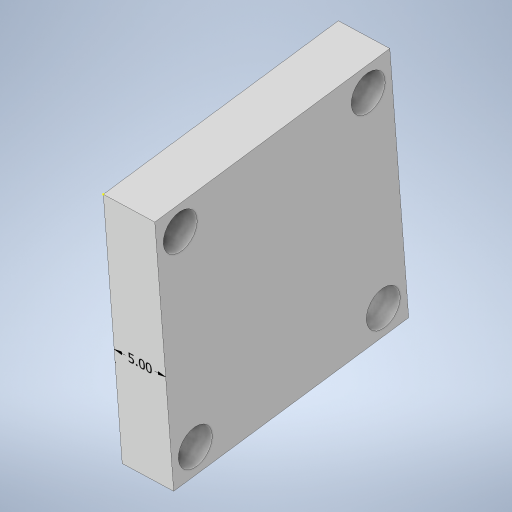
# Autodesk Inventor part: Plate_5mmforPrint
Saved by Autodesk Inventor 2024 (Build 280153000, 153)
## iProperties
Created: 2023-11-01
Part Number: Plate_5mmforPrint
Material: 一般
Document SubType Name: Modeling
Designer: jwith
Density: 1 g/cm^3
Appearance: 既定
Author: jwith
Autodesk Inventor part; units mm, degrees
ref_plane "YZ Plane" through (0, 0, 0) normal (1, 0, 0) x (0, 1, 0)
ref_plane "XZ Plane" through (0, 0, 0) normal (0, 1, 0) x (-1, 0, 0)
ref_plane "XY Plane" through (0, 0, 0) normal (0, 0, 1) x (1, 0, 0)
sketch "スケッチ1" plane through (0, 0, 0) normal (0, 1, 0) x (-1, 0, 0)
  line L0 (0, 0) -> (25, 0)
  line L1 (25, 0) -> (25, -25)
  line L2 (25, -25) -> (0, -25)
  line L3 (0, -25) -> (0, 0)
  dimension "d0" = 25
  dimension "d1" = 25
  constraints: 8 end point, 2 parallel, 1 horizontal, 1 perpendicular
  measures "d0" distance of L0.end L1.end
  measures "d1" distance of L1.end L2.end
extrude "押し出し1" add sketch "スケッチ1" against normal blind 5
sketch "スケッチ2" plane through (0, 0, 0) normal (0, 1, 0) x (1, 0, 0)
  line L0 (0, 25) -> (-25, 25) projected
  line L1 (0, 0) -> (0, 25) projected
  point P0 (-2.5, 22.5)
  point P1 (-22.5, 22.5)
  point P2 (-22.5, 2.5)
  point P3 (-2.5, 2.5)
  dimension "d4" = 20
  dimension "d5" = 20
  dimension "d6" = 20
  dimension "d7" = 20
  dimension "d8" = 2.5
  dimension "d9" = 2.5
  dimension "d10" = 2.5
  dimension "d11" = 2.5
  measures "d4" distance of point (-2.5, 22.5) point (-22.5, 22.5)
  measures "d5" distance of point (-2.5, 2.5) point (-2.5, 22.5)
  measures "d6" distance of point (-2.5, 2.5) point (-22.5, 2.5)
  measures "d7" distance of point (-22.5, 2.5) point (-22.5, 22.5)
  measures "d8" distance from line of L0 point (-22.5, 22.5)
  measures "d9" distance from line of L0 point (-2.5, 22.5)
  measures "d10" distance from line of L1 point (-2.5, 22.5)
  measures "d11" distance from line of L1 point (-2.5, 2.5)
hole "穴1" at (-2.5, 0, -22.5) at (-22.5, 0, -22.5) at (-22.5, 0, -2.5) at (-2.5, 0, -2.5) direction (0, -1, 0) diameter 3.6 end through all
sketch "スケッチ3" plane through (0, -5, 0) normal (0, -1, 0) x (1, 0, 0)
  point P0 (0, 0)
